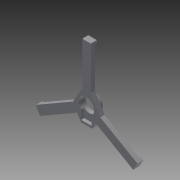
# Autodesk Inventor part: BaseVentosa
Saved by Autodesk Inventor 2014 SP1 (Build 180222100, 222)
## iProperties
Created: 2014-03-05
Part Number: BaseVentosa
Material: Genérico
Document SubType Name: Modeling
Designer: Gregorio
Density: 1 g/cm^3
Appearance: Valor por defecto
Author: Gregorio
Autodesk Inventor part; units mm, degrees
ref_plane "YZ Plane" through (0, 0, 0) normal (1, 0, 0) x (0, 1, 0)
ref_plane "XZ Plane" through (0, 0, 0) normal (0, 1, 0) x (-1, 0, 0)
ref_plane "XY Plane" through (0, 0, 0) normal (0, 0, 1) x (1, 0, 0)
sketch "Boceto1" plane through (0, 0, 0) normal (0, 1, 0) x (-1, 0, 0)
  circle A0 centre (6.15, 17.029) radius 9
  dimension "d2" = 18
  constraints: 1 centre point
  measures "d2" diameter of A0
sketch "Boceto2" plane through (0, 0, 0) normal (0, 1, 0) x (-1, 0, 0)
  line L0 (6, -14) -> (-20.8468, 32.5)
  line L1 (-20.8468, 32.5) -> (32.8468, 32.5)
  line L2 (32.8468, 32.5) -> (6, -14)
  point P0 (0, 0)
  point P1 (6, 17)
  constraints: 6 end point, 7 other
extrude "Extrusión1" add sketch "Boceto2" along normal blind 5
extrude "Extrusión2" cut sketch "Boceto1" along normal blind 5
sketch "Boceto3" plane through (0, 0, 0) normal (0, -1, 0) x (1, 0, 0)
  circle A0 centre (-6.15, 17.029) radius 9 projected
  line L0 (-12.3, 23.6) -> (0, 23.6)
  line L1 (0, 23.6) -> (0, 0)
  line L2 (0, 0) -> (-12.3, 0)
  line L3 (-12.3, 0) -> (-12.3, 23.6)
  point P0 (0, 0)
  point P1 (-6.15, 23.6)
  dimension "d7" = 12.3
  dimension "d8" = 23.6
  constraints: 8 end point, 2 parallel, 1 horizontal, 1 midpoint, 1 perpendicular, 1 vertical alignment, 2 other
  measures "d7" distance of L1.end L2.end
  measures "d8" distance of L0.end L1.end
extrude "Extrusión3" cut sketch "Boceto3" against normal blind 3.5 contours L1 A0 L3 L0 | L1 L2 L3 A0
sketch "Boceto4" plane through (0, 5, 0) normal (0, 1, 0) x (1, 0, 0)
  circle A0 centre (-6.15, -17.029) radius 9 projected
  circle A1 centre (-6.15, -17.029) radius 11.0617
  point P0 (0, 0)
  constraints: 1 centre point, 1 coincident
extrude "Extrusión4" add sketch "Boceto4" along normal blind 3
sketch "Boceto5" plane through (-32.8468, 0, 32.5) normal (0, 0, 1) x (1, 0, 0)
  line L0 (53.6936, 0) -> (0, 0) projected
  line L1 (0, 5) -> (53.6936, 5) projected
  line L2 (21.8468, 5) -> (31.8468, 5)
  line L3 (31.8468, 5) -> (31.8468, 0)
  line L4 (31.8468, 0) -> (21.8468, 0)
  line L5 (21.8468, 0) -> (21.8468, 5)
  point P0 (32.8468, 0)
  point P1 (26.8468, 0)
  point P2 (26.8468, 0)
  dimension "d13" = 10
  constraints: 8 end point, 2 midpoint, 2 parallel, 2 point on line, 1 coincident, 1 horizontal, 1 perpendicular
  measures "d13" distance of L3.end L4.end
extrude "Extrusión5" add sketch "Boceto5" along normal blind 50
sketch "Boceto6" plane through (-32.8468, 0, 32.5) normal (-0.8660254, 0, -0.5) x (-0.5, 0, 0.8660254)
  line L0 (-53.6936, 5) -> (0, 5) projected
  line L1 (-31.8468, 5) -> (-21.8468, 5)
  line L2 (-21.8468, 5) -> (-21.8468, 0)
  line L3 (-21.8468, 0) -> (-31.8468, 0)
  line L4 (-31.8468, 0) -> (-31.8468, 5)
  point P0 (-44.5692, 0)
  point P1 (-26.8468, 5)
  point P2 (-26.8468, 5)
  dimension "d16" = 10
  dimension "d17" = 5
  constraints: 8 end point, 2 midpoint, 2 parallel, 1 coincident, 1 horizontal, 1 perpendicular, 1 point on line
  measures "d16" distance of L2.end L3.end
  measures "d17" distance of L1.end L2.end
extrude "Extrusión6" add sketch "Boceto6" along normal blind 50
sketch "Boceto7" plane through (-6, 0, -14) normal (0.8660254, 0, -0.5) x (-0.5, 0, -0.8660254)
  line L0 (0, 0) -> (-53.6936, 0) projected
  line L1 (-53.6936, 5) -> (0, 5) projected
  line L2 (-31.8468, 5) -> (-21.8468, 5)
  line L3 (-21.8468, 5) -> (-21.8468, 0)
  line L4 (-21.8468, 0) -> (-31.8468, 0)
  line L5 (-31.8468, 0) -> (-31.8468, 5)
  point P0 (-15.1244, 0)
  point P1 (-26.8468, 5)
  point P2 (-26.8468, 5)
  dimension "d20" = 10
  constraints: 8 end point, 2 midpoint, 2 parallel, 2 point on line, 1 coincident, 1 horizontal, 1 perpendicular
  measures "d20" distance of L3.end L4.end
extrude "Extrusión7" add sketch "Boceto7" along normal blind 50
chamfer "Chaflán1" distance 13.25 angle 45 1 edges at (-6, 2.5, -14)
sketch "Boceto8" plane through (0, 0, 0) normal (0, -1, 0) x (1, 0, 0)
  line L0 (9.9234, 13.5801) -> (20.8468, 32.5) projected
  line L1 (20.8468, 32.5) -> (-1, 32.5) projected
  line L2 (-11, 32.5) -> (-32.8468, 32.5) projected
  line L3 (-32.8468, 32.5) -> (-21.9234, 13.5801) projected
  line L4 (-16.9234, 4.9199) -> (-12.625, -2.5252) projected
  line L5 (-21.9234, 13.5801) -> (-11, 32.5)
  line L6 (-11, 32.5) -> (-31.0383, 44.0691)
  line L7 (-31.0383, 44.0691) -> (-41.9617, 25.1492)
  line L8 (-41.9617, 25.1492) -> (-21.9234, 13.5801)
  line L9 (-1, 32.5) -> (9.9234, 13.5801)
  line L10 (9.9234, 13.5801) -> (33.1734, 27.0035)
  line L11 (33.1734, 27.0035) -> (22.25, 45.9234)
  line L12 (22.25, 45.9234) -> (-1, 32.5)
  constraints: 16 end point, 6 parallel, 2 perpendicular
extrude "Extrusión8" cut sketch "Boceto8" against normal blind 5 contours L9 L1 L0 | L5 L3 L2
sketch "Boceto9" plane through (0, 5, 0) normal (0, 1, 0) x (1, 0, 0)
  line L0 (48.2247, 20.0801) -> (53.2247, 11.4199) projected
  line L1 (-16.9234, -4.9199) -> (-60.2247, 20.0801) projected
  line L2 (-11, -32.5) -> (-11, -82.5) projected
  line L3 (-60.2247, 20.0801) -> (-57.6266, 18.5801)
  line L4 (-57.6266, 18.5801) -> (-62.6266, 9.9199)
  line L5 (-62.6266, 9.9199) -> (-65.2247, 11.4199)
  line L6 (-65.2247, 11.4199) -> (-60.2247, 20.0801)
  line L7 (48.2247, 20.0801) -> (53.2247, 11.4199)
  line L8 (53.2247, 11.4199) -> (50.6266, 9.9199)
  line L9 (50.6266, 9.9199) -> (45.6266, 18.5801)
  line L10 (45.6266, 18.5801) -> (48.2247, 20.0801)
  line L11 (-1, -82.5) -> (-11, -82.5)
  line L12 (-11, -82.5) -> (-11, -79.5)
  line L13 (-11, -79.5) -> (-1, -79.5)
  line L14 (-1, -79.5) -> (-1, -82.5)
  point P0 (0, 0)
  dimension "d31" = 3
  dimension "d32" = 3
  constraints: 24 end point, 7 equal length, 4 perpendicular, 1 point on line
  measures "d31" distance of L4.end L5.end
  measures "d32" distance of L2.end L12.end
extrude "Extrusión9" add sketch "Boceto9" along normal blind 2
